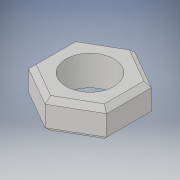
# Autodesk Inventor part: M8_Nut
Saved by Autodesk Inventor 2019 (Build 230136000, 136)
## iProperties
Created: 2019-10-16
Part Number: M8_Nut
Material: Generic
Document SubType Name: Modeling
Designer: 19879326
Density: 1 g/cm^3
Appearance: Default
Author: 19879326
Autodesk Inventor part; units mm, degrees
ref_plane "YZ Plane" through (0, 0, 0) normal (1, 0, 0) x (0, 1, 0)
ref_plane "XZ Plane" through (0, 0, 0) normal (0, 1, 0) x (-1, 0, 0)
ref_plane "XY Plane" through (0, 0, 0) normal (0, 0, 1) x (1, 0, 0)
sketch "Sketch1" plane through (0, 0, 0) normal (0, 1, 0) x (-1, 0, 0)
  line L0 (6.5, -3.7528) -> (0, -7.5056)
  line L1 (0, -7.5056) -> (-6.5, -3.7528)
  line L2 (-6.5, -3.7528) -> (-6.5, 3.7528)
  line L3 (-6.5, 3.7528) -> (0, 7.5056)
  line L4 (0, 7.5056) -> (6.5, 3.7528)
  line L5 (6.5, 3.7528) -> (6.5, -3.7528)
  circle A0 centre (0, 0) radius 4
  point P0 (6.5, 0)
  dimension "d0" = 13
  dimension "d3" = 8
  constraints: 12 end point, 2 coincident, 1 centre point, 1 horizontal alignment, 1 midpoint, 13 other
  measures "d0" distance between parallel lines of L2 L5
  measures "d3" diameter of A0
extrude "Extrusion1" add sketch "Sketch1" along normal blind 5
chamfer "Chamfer1" distance 0.8 angle 45 12 edges at (-3.25, 5, 5.6292) (-6.5, 5, 0) (-3.25, 5, -5.6292) (3.25, 5, -5.6292) (6.5, 5, 0) (3.25, 5, 5.6292) (-3.25, 0, 5.6292) (3.25, 0, 5.6292) (6.5, 0, 0) (3.25, 0, -5.6292) (-3.25, 0, -5.6292) (-6.5, 0, 0)
body "Solid1"
